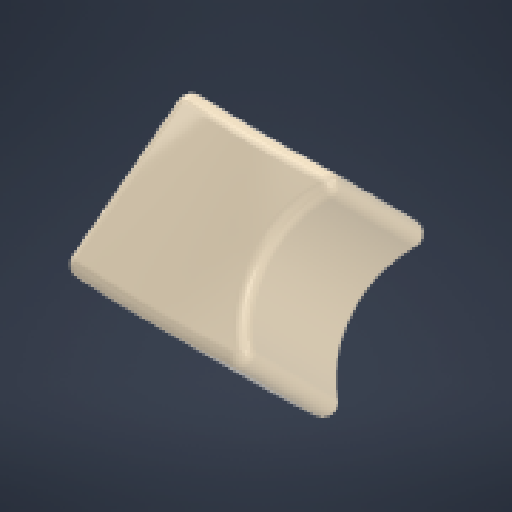
# Autodesk Inventor part: SPACER_ROLLER_CR_BEARING,REV-ENG
Saved by Autodesk Inventor 2026.2 (Build 302298010, 298A)
## iProperties
Created: 2026-03-05
Part Number: SPACER_ROLLER_CR_BEARING,REV-ENG
Material: Iglidur,V400
Document SubType Name: Modeling
Designer: 4aida
Density: 1.49472 g/cm^3
Appearance: Smooth - Light Beige
Author: 4aida
Autodesk Inventor part; units mm, degrees
ref_plane "YZ Plane" through (0, 0, 0) normal (1, 0, 0) x (0, 1, 0)
ref_plane "XZ Plane" through (0, 0, 0) normal (0, 1, 0) x (-1, 0, 0)
ref_plane "XY Plane" through (0, 0, 0) normal (0, 0, 1) x (1, 0, 0)
sketch "Sketch1" plane through (0, 0, 0) normal (1, 0, 0) x (0, 1, 0)
  line L0 (2.4749, 25) -> (0, 27.4749)
  line L1 (0, 27.4749) -> (-2.4749, 25)
  line L2 (-2.4749, 25) -> (0, 22.5251)
  line L3 (0, 22.5251) -> (2.4749, 25)
  line L4 (0, 0) -> (2.4749, 0)
  line L5 (0, 27.4749) -> (0, 22.5251) construction
  line L6 (-2.8284, 25) -> (0, 27.8284) construction
  line L7 (0, 27.8284) -> (2.8284, 25) construction
  line L8 (2.8284, 25) -> (0, 22.1716) construction
  line L9 (0, 22.1716) -> (-2.8284, 25) construction
  line L10 (-2.8284, 25) -> (2.8284, 25) construction
  line L11 (0, 27.8284) -> (0, 22.1716) construction
  point P0 (0, 25)
  point P1 (0, 25)
  dimension "d0" = 3.5
  dimension "d1" = 3.5
  dimension "d4" = 50
  dimension "d26" = 4
  dimension "d27" = 55.6568
  dimension "d28" = 5.6569
  constraints: 24 end point, 5 midpoint, 4 parallel, 3 perpendicular, 2 vertical alignment, 1 horizontal, 1 point on line, 1 vertical
  measures "d0" distance of L0.start L0.end
  measures "d1" distance of L2.end L0.start
  measures "d4" diameter of point (0, 25) L4
  measures "d26" distance between parallel lines of L6 L8
  measures "d27" diameter of L6.end L4
  measures "d28" distance of L8.end L6.end
revolve "Revolution1" add sketch "Sketch1" angle 15 mid plane about axis through (0, 0, 0) along (0, 1, 0)
ref_plane "Work Plane4" through (3.2632, 2.4749, 24.7861) normal (0.092296, 0.7071068, 0.7010574) x (0.092296, -0.7071068, 0.7010574)
ref_plane "Work Plane5" through (-3.5862, 0, 27.2398) normal (0.092296, 0.7071068, -0.7010574) x (0.092296, -0.7071068, -0.7010574)
sketch "Sketch4" plane through (3.2632, 2.4749, 24.7861) normal (0.092296, 0.7071068, 0.7010574) x (0.092296, -0.7071068, 0.7010574)
  line L0 (3.5, 0) -> (0, 0) projected
  circle A0 centre (1.75, 0) radius 2.0625
  point P0 (-15.9277, 0)
  dimension "d19" = 4.125
  constraints: 1 centre point, 1 midpoint
  measures "d19" diameter of A0
extrude "Extrusion3" cut sketch "Sketch4" against normal through all
sketch "Sketch5" plane through (-3.5862, 0, 27.2398) normal (0.092296, 0.7071068, -0.7010574) x (0.092296, -0.7071068, -0.7010574)
  line L0 (3.5, 0) -> (0, 0) projected
  circle A0 centre (1.75, 0) radius 2.0625
  point P0 (19.4277, 0)
  dimension "d22" = 4.125
  constraints: 1 centre point, 1 midpoint
  measures "d22" diameter of A0
extrude "Extrusion4" cut sketch "Sketch5" along normal through all
fillet "Fillet3" radius 0.25 12 edges at (0.0271, 2.4749, 25) (0, 0, 22.5251) (0, 0, 27.4749) (-0.0271, -2.4749, 25) (-1.3712, -1.2257, 26.2133) (-2.0436, -1.2374, 23.6745) (-1.0473, 1.2504, 23.7524) (-2.313, 1.2375, 26.1353) (1.3712, 1.2257, 26.2133) (2.313, -1.2375, 26.1353) (1.0473, -1.2504, 23.7524) (2.0436, 1.2374, 23.6745)
equation "\"d1\" = d0"
body "Solid1"
